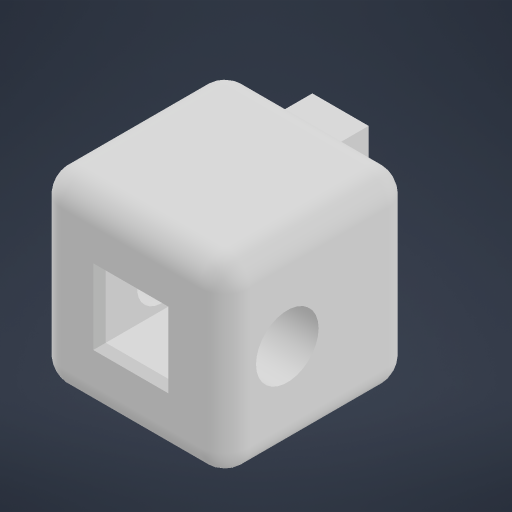
# Autodesk Inventor part: Hole_TestFits
Saved by Autodesk Inventor 2024 (Build 280153000, 153)
## iProperties
Created: 2023-07-01
Part Number: Hole_TestFits
Material: Generic
Document SubType Name: Modeling
Designer: User
Density: 1 g/cm^3
Appearance: Default
Author: User
Autodesk Inventor part; units mm, degrees
ref_plane "YZ Plane" through (0, 0, 0) normal (1, 0, 0) x (0, 1, 0)
ref_plane "XZ Plane" through (0, 0, 0) normal (0, 1, 0) x (-1, 0, 0)
ref_plane "XY Plane" through (0, 0, 0) normal (0, 0, 1) x (1, 0, 0)
sketch "Sketch14" plane through (0, 0, 0) normal (0, 0, 1) x (1, 0, 0)
  line L0 (0, 0) -> (-15, 0)
  line L1 (-15, 0) -> (-15, 15)
  line L2 (-15, 15) -> (0, 15)
  line L3 (0, 15) -> (0, 0)
  line L4 (-5, 5) -> (-10, 5)
  line L5 (-10, 5) -> (-10, 10)
  line L6 (-10, 10) -> (-5, 10)
  line L7 (-5, 10) -> (-5, 5)
  dimension "d71" = 15
  dimension "d72" = 15
  dimension "d73" = 5
  dimension "d74" = 5
  constraints: 16 end point, 4 parallel, 2 horizontal, 2 perpendicular
  measures "d71" distance of L1.end L2.end
  measures "d72" distance of L0.end L1.end
  measures "d73" distance of L5.end L6.end
  measures "d74" distance of L4.end L5.end
extrude "Extrusion9" add sketch "Sketch14" along normal blind 15 contours L0 L1 L2 L3 | L4 L5 L6 L7
sketch "Sketch16" plane through (0, 0, 15) normal (0, 0, 1) x (1, 0, 0)
  line L0 (-5, 5) -> (-10, 5)
  line L1 (-10, 5) -> (-10, 10)
  line L2 (-10, 10) -> (-5, 10)
  line L3 (-5, 10) -> (-5, 5)
  point P0 (0, 0)
  dimension "d84" = 5
  dimension "d85" = 5
  constraints: 8 end point, 2 parallel, 1 horizontal, 1 perpendicular
  measures "d84" distance of L1.end L2.end
  measures "d85" distance of L0.end L1.end
extrude "Extrusion11" cut sketch "Sketch16" against normal blind 10
chamfer "Chamfer5" distance 0.5 angle 45 4 edges at (-7.5, 10, 15) (-10, 7.5, 15) (-7.5, 5, 15) (-5, 7.5, 15)
sketch "Sketch19" plane through (0, 0, 0) normal (0, 0, -1) x (-1, 0, 0)
  line L0 (12, 12) -> (7.5, 12)
  line L1 (7.5, 12) -> (7.5, 7.5)
  line L2 (7.5, 7.5) -> (12, 7.5)
  line L3 (12, 7.5) -> (12, 12)
  point P0 (0, 0)
  point P1 (15, 15)
  dimension "d142" = 4.5
  dimension "d143" = 4.5
  constraints: 8 end point, 2 parallel, 1 horizontal, 1 perpendicular
  measures "d142" distance of L2.end L1.end
  measures "d143" distance of L1.end L0.end
extrude "Extrusion13" add sketch "Sketch19" along normal blind 5
chamfer "Chamfer10" distance 1 angle 45 4 edges at (-9.75, 12, -5) (-12, 9.75, -5) (-9.75, 7.5, -5) (-7.5, 9.75, -5)
sketch "Sketch22" plane through (-15, 0, 0) normal (-1, 0, 0) x (0, 0, 1)
  point P0 (0, 0)
  point P1 (10, 7.5)
hole "Hole9" at (-15, 7.5, 10) direction (1, 0, 0) diameter 4 depth 6 counterbore diameter 5 counterbore depth 4.5
sketch "Sketch23" plane through (0, 0, 0) normal (1, 0, 0) x (0, 0, -1)
  point P0 (0, 0)
  point P1 (-10, 7.5)
hole "Hole10" at (0, 7.5, 10) direction (-1, 0, 0) diameter 4 depth 6 counterbore diameter 5 counterbore depth 4.5
fillet "Fillet1" radius 2 12 edges at (-15, 15, 7.5) (-15, 7.5, 0) (-15, 0, 7.5) (-15, 7.5, 15) (0, 7.5, 15) (-7.5, 15, 15) (0, 15, 7.5) (-7.5, 15, 0) (-7.5, 0, 15) (0, 7.5, 0) (0, 0, 7.5) (-7.5, 0, 0)
body "Solid4"
